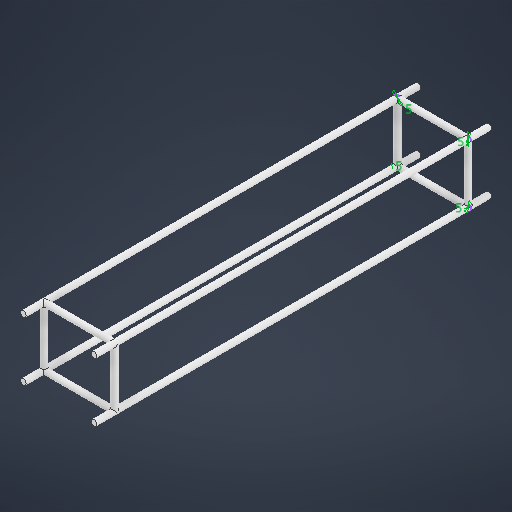
# Autodesk Inventor part: RCPlaneSkeletonModel1
Saved by Autodesk Inventor 2026.1 (Build 301233000, 233)
## iProperties
Created: 2026-02-24
Part Number: RCPlaneSkeletonModel1
Material: PC/ABS Plastic
Document SubType Name: Modeling
Designer: morri
Density: 1.1 g/cm^3
Appearance: Smooth - White
Mass: 37.6897 g
Surface Area: 272.93 cm^2
Volume: 34.2633 cm^3
Author: morri
Autodesk Inventor part; units mm, degrees
ref_plane "YZ Plane" through (0, 0, 0) normal (1, 0, 0) x (0, 1, 0)
ref_plane "XZ Plane" through (0, 0, 0) normal (0, 1, 0) x (-1, 0, 0)
sketch "Sketch1" plane through (0, 0, 0) normal (0, 0, 1) x (1, 0, 0)
  circle A0 centre (0, 0) radius 2.5
  circle A1 centre (0, 50) radius 2.5
  circle A2 centre (60, 50) radius 2.5
  circle A3 centre (60, 0) radius 2.5
  dimension "d0" = 5
  dimension "d11" = 5
  dimension "d12" = 5
  dimension "d13" = 5
  constraints: 4 centre point, 1 coincident
  measures "d0" diameter of A0
  measures "d11" diameter of A1
  measures "d12" diameter of A2
  measures "d13" diameter of A3
sketch "Sketch2" plane through (0, 0, 0) normal (1, 0, 0) x (0, 1, 0)
  circle A0 centre (0, 0) radius 2.5
  circle A1 centre (50, 0) radius 2.5
  circle A2 centre (0, 300) radius 2.5
  circle A3 centre (50, 300) radius 2.5
  dimension "d1" = 5
  dimension "d27" = 5
  dimension "d35" = 5
  dimension "d36" = 5
  constraints: 4 centre point, 1 coincident
  measures "d1" diameter of A0
  measures "d27" diameter of A1
  measures "d35" diameter of A2
  measures "d36" diameter of A3
sketch "Sketch3" plane through (0, 0, 0) normal (0, 1, 0) x (-1, 0, 0)
  circle A0 centre (0, 0) radius 2.5
  circle A1 centre (-60, 0) radius 2.5
  circle A2 centre (0, 300) radius 2.5
  circle A3 centre (-60, 300) radius 2.5
  dimension "d2" = 5
  dimension "d31" = 5
  dimension "d42" = 5
  dimension "d43" = 5
  constraints: 4 centre point, 1 coincident
  measures "d2" diameter of A0
  measures "d31" diameter of A1
  measures "d42" diameter of A2
  measures "d43" diameter of A3
extrude "LongBL" add sketch "Sketch1" along normal blind 300 contours A0
extrude "SideBB" add sketch "Sketch3" along normal blind 50 contours A0
extrude "UpBL" add sketch "Sketch2" along normal blind 60 contours A0
extrude "LongBR" add sketch "Sketch1" along normal blind 300 contours A3
extrude "LongTL" add sketch "Sketch1" along normal blind 300 contours A1
extrude "LongTR" add sketch "Sketch1" along normal blind 300 contours A2
extrude "Extrusion9" add sketch "Sketch2" along normal blind 60 contours A1
extrude "Extrusion10" add sketch "Sketch3" along normal blind 50 contours A1
extrude "Extrusion11" add sketch "Sketch2" along normal blind 60 contours A3
extrude "Extrusion12" add sketch "Sketch2" along normal blind 60 contours A2
extrude "Extrusion13" add sketch "Sketch3" along normal blind 50 contours A3
extrude "Extrusion14" add sketch "Sketch3" along normal blind 50 contours A2
ref_plane "Work Plane3" through (-2.5, 0, 300) normal (0, 0, 1) x (1, 0, 0)
sketch "Sketch5" plane through (-2.5, 0, 300) normal (0, 0, 1) x (1, 0, 0)
  arc A0 (4.2678, 1.7678) -> (0, 0) centre (2.5, 0) ccw projected
  line L0 (0, 0) -> (2.5, 0) projected
  circle A1 centre (2.5, 0) radius 2.5
  line L1 (2.5, 50) -> (2.5, 52.5) projected
  circle A2 centre (2.5, 50) radius 2.5
  line L2 (62.5, 50) -> (60, 47.5) projected
  circle A3 centre (62.5, 50) radius 2.5
  arc A4 (60.7322, 1.7678) -> (62.5, -2.5) centre (62.5, 0) ccw projected
  circle A5 centre (62.5, 0) radius 2.5
  point P0 (60.7322, 48.2322)
  dimension "d48" = 5
  dimension "d49" = 5
  dimension "d50" = 5
  dimension "d51" = 5
  constraints: 3 centre point, 2 coincident, 1 horizontal alignment, 2 other
  measures "d49" diameter of A2
  measures "d50" diameter of A3
  measures "d51" diameter of A5
extrude "FTLConnect" add sketch "Sketch5" along normal blind 17.5 contours A2
sketch "Sketch7" plane through (-2.5, 0, 300) normal (0, 0, 1) x (1, 0, 0)
  arc A0 (0, 0) -> (2.5, -2.5) centre (2.5, 0) ccw projected
  line L0 (2.5, -2.5) -> (2.5, 0) projected
  circle A1 centre (2.5, 0) radius 2.5
  line L1 (65, 50) -> (62.5, 50) projected
  circle A2 centre (62.5, 50) radius 2.5
  circle A3 centre (62.5, 0) radius 2.5
  constraints: 1 centre point, 1 coincident, 1 horizontal alignment, 1 vertical alignment, 4 other
extrude "FTRConnect" add sketch "Sketch7" along normal blind 17.5 contours A2
sketch "Sketch8" plane through (-2.5, 0, 300) normal (0, 0, 1) x (1, 0, 0)
  line L0 (2.5, -2.5) -> (2.5, 0) projected
  circle A0 centre (2.5, 0) radius 2.5
  dimension "d56" = 5
  constraints: 1 centre point, 1 coincident
  measures "d56" diameter of A0
extrude "FBLConnect" add sketch "Sketch8" along normal blind 17.5
sketch "Sketch9" plane through (-2.5, 0, 300) normal (0, 0, 1) x (1, 0, 0)
  circle A0 centre (62.5, 0) radius 2.5
  point P0 (2.5, 0)
  dimension "d59" = 5
  constraints: 1 centre point
  measures "d59" diameter of A0
extrude "FBRConnect" add sketch "Sketch9" along normal blind 17.5
extrude "BTRConnect" add sketch "Sketch1" against normal blind 17.5 contours A2
extrude "BTLConnect" add sketch "Sketch1" against normal blind 17.5 contours A1
extrude "BBRConnect" add sketch "Sketch1" against normal blind 17.5 contours A3
extrude "BBLConnect" add sketch "Sketch1" against normal blind 17.5 contours A0
body "Solid1"
